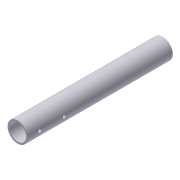
# Autodesk Inventor part: FE-00005-02
Saved by Autodesk Inventor 2012 (Build 160160000, 160)
## iProperties
Company: FIRST
Created: 2008-05-25
Part Number: FE-00005-02
Document SubType Name: Modeling
Designer: dfoster
Density: 1 g/cm^3
Description: Connecting Tube - Field Rail
Mass: 129.955 g
Surface Area: 738.364 cm^2
Volume: 129.955 cm^3
Material: Default
Title: Connecting Tube - Field Rail
Author: dfoster
Autodesk Inventor part; units mm, degrees
ref_plane "XZ Plane" through (0, 0, 0) normal (0, 1, 0) x (-1, 0, 0)
ref_plane "XY Plane" through (0, 0, 0) normal (0, 0, 1) x (1, 0, 0)
sketch "Sketch1" plane through (0, 0, 0) normal (0, 0, 1) x (1, 0, 0)
  circle A0 centre (0, 0) radius 21.0312
  circle A1 centre (0, 0) radius 17.4625
  dimension "d0" = 42.0624
  dimension "d1" = 34.925
  constraints: 2 centre point, 1 coincident
  measures "d0" diameter of A0
  measures "d1" diameter of A1
extrude "Extrusion1" add sketch "Sketch1" along normal blind 301.625
ref_plane "Work Plane2" through (0, 0, 0) normal (1, 0, 0) x (0, 0, 1)
sketch "Sketch3" plane through (0, 0, 0) normal (1, 0, 0) x (0, 0, 1)
  line L0 (301.625, 17.4625) -> (301.625, -17.4625) projected
  line L1 (301.625, 21.0312) -> (301.625, -21.0312) projected
  line L2 (-60.325, 0) -> (361.95, 0) projected
  circle A0 centre (276.225, 0) radius 3.175
  dimension "d10" = 6.35
  dimension "d11" = 25.4
  constraints: 1 centre point, 1 point on line
  measures "d10" diameter of A0
  measures "d11" distance from line of L0 A0.centre
extrude "Extrusion3" cut sketch "Sketch3" along normal blind 381
pattern_linear "Rectangular Pattern1" count 2 spacing 50.8 along (0, 0, -1) of "Extrusion3"
body "Solid1"
